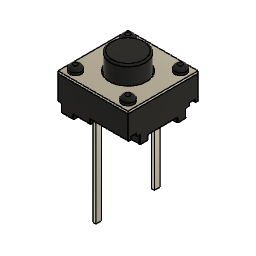
6x6x5 (Autodesk Fusion 360 design; units mm, degrees)
Autodesk Fusion 360 part; units mm, degrees
note: some values were not read from the file. Chosen so that the rebuilt part matches the saved one: which pieces of a blend or face edit are solid.
sketch "Sketch1" plane through (0, 0, 0) normal (0, 0, 1) x (1, 0, 0)
  line L0 (3, -3) -> (-3, -3)
  line L1 (-3, -3) -> (-3, 3)
  line L2 (-3, 3) -> (3, 3)
  line L3 (3, 3) -> (3, -3)
  line L4 (3, -3) -> (-3, 3) construction
  line L5 (-3, -3) -> (3, 3) construction
  dimension "d1" = 6
  dimension "d2" = 6
  constraint horizontal L0
  constraint perpendicular L0 L1
  constraint parallel L0 L2
  constraint parallel L1 L3
  constraint coincident L4 origin
  constraint coincident L5 origin
  measures "d1" distance of L1.end L2.end
  measures "d2" distance of L0.end L1.end
extrude "Extrude1" add sketch "Sketch1" along normal blind 2.8 makes body 1
extrude "Extrude2" add 1 faces at (-1, -1, 2.8) along direction (0, 0, 1) blind 0.2 separate body on bodies 1 makes body 2
sketch "Sketch2" plane through (0, 0, 3) normal (0, 0, 1) x (-1, 0, 0)
  line L0 (-3, -3) -> (3, -3)
  line L1 (3, -3) -> (3, 3)
  line L2 (3, 3) -> (-3, 3)
  line L3 (-3, 3) -> (-3, -3)
  circle A0 centre (2.25, -2.25) radius 0.5
  circle A1 centre (0, 0) radius 1.5
  circle A2 centre (0, 0) radius 1.6
  dimension "d7" = 1
  dimension "d8" = 0.75
  dimension "d9" = 0.75
  dimension "d10" = 3
  dimension "d23" = 3.2
  constraint coincident A1.centre A2.centre
  constraint concentric A1 A2
  measures "d7" diameter of A0
  measures "d8" distance of L0 A0.centre
  measures "d9" distance of L1 A0.centre
  measures "d10" diameter of A1
  measures "d23" diameter of A2
extrude "Extrude3" add sketch "Sketch2" along normal blind 0.5 contours A0 bodies 2
extrude "Extrude4" add sketch "Sketch2" along normal blind 1.5 contours A1 bodies 2
fillet "Fillet1" radius 0.3 1 edges at (-1.7838, 2.4308, 3.5) on bodies 2
mirror "Mirror1" about plane through (0, 0, 0) normal (1, 0, 0) of "Extrude3", "Fillet1"
mirror "Mirror2" about plane through (0, 0, 0) normal (0, 1, 0) of "Extrude3", "Fillet1", "Mirror1"
fillet "Fillet2" radius 0.15 1 edges at (1.3985, 0.5424, 4.5) on bodies 2
extrude "Extrude5" cut sketch "Sketch2" against normal blind 0.2 contours A2 bodies 2 makes body 3 at (-0.0399, 2.5318, 2.8)
sketch "Sketch3" plane through (3, 0, 0) normal (1, 0, 0) x (0, 1, 0)
  line L0 (-3, 0) -> (3, 0)
  line L1 (3, 0) -> (3, 2.8)
  line L2 (3, 2.8) -> (-3, 2.8)
  line L3 (-3, 2.8) -> (-3, 0)
  line L4 (-2, 0) -> (-1.25, 0)
  line L5 (-1.25, 0) -> (-1.25, 0.75)
  line L6 (-1.25, 0.75) -> (-2, 0.75)
  line L7 (-2, 0.75) -> (-2, 0)
  line L8 (-2.75, 0.75) -> (-2.25, 0.75)
  line L9 (-2.25, 0.75) -> (-2.25, 1)
  line L10 (-2.25, 1) -> (-2.75, 1)
  line L11 (-2.75, 1) -> (-2.75, 0.75)
  line L12 (-2, 0.75) -> (-3, 0.75)
  line L13 (2, 0) -> (1.25, 0)
  line L14 (1.25, 0) -> (1.25, 0.75)
  line L15 (1.25, 0.75) -> (2, 0.75)
  line L16 (2, 0.75) -> (2, 0)
  line L17 (-1.25, 0.75) -> (1.25, 0.75)
  line L18 (1.25, 0.75) -> (1.25, 0.375)
  line L19 (1.25, 0.375) -> (-1.25, 0.375)
  line L20 (-1.25, 0.375) -> (-1.25, 0.75)
  line L21 (2, 0.75) -> (3, 0.75)
  line L22 (2.75, 0.75) -> (2.25, 0.75)
  line L23 (2.25, 0.75) -> (2.25, 1)
  line L24 (2.25, 1) -> (2.75, 1)
  line L25 (2.75, 1) -> (2.75, 0.75)
  dimension "d26" = 0.75
  dimension "d27" = 0.75
  dimension "d28" = 1
  dimension "d29" = 0.5
  dimension "d30" = 0.25
  dimension "d31" = 0.25
  dimension "d32" = 0.75
  dimension "d33" = 0.75
  dimension "d34" = 1
  dimension "d35" = 0.5
  dimension "d36" = 0.25
  dimension "d37" = 0.25
  constraint horizontal L4
  constraint vertical L5
  constraint horizontal L6
  constraint vertical L7
  constraint coincident L0 L4.start
  constraint horizontal L8
  constraint vertical L9
  constraint horizontal L10
  constraint vertical L11
  constraint coincident L3 L12.end
  constraint perpendicular L3 L12
  constraint horizontal L13
  constraint vertical L14
  constraint horizontal L15
  constraint vertical L16
  constraint coincident L0 L13.start
  constraint horizontal L17
  constraint vertical L18
  constraint horizontal L19
  constraint vertical L20
  constraint midpoint L14 L18.end
  constraint coincident L1 L21.end
  constraint perpendicular L1 L21
  constraint horizontal L22
  constraint vertical L23
  constraint horizontal L24
  constraint vertical L25
  constraint coincident L21 L22.start
  measures "d26" distance of L4.start L4.end
  measures "d27" distance of L4.start L6.end
  measures "d28" distance of L3 L7
  measures "d29" distance of L8.start L8.end
  measures "d30" distance of L8.start L10.end
  measures "d31" distance of L3 L11
  measures "d32" distance of L13.start L13.end
  measures "d33" distance of L13.start L15.end
  measures "d34" distance of L1 L16
  measures "d35" distance of L22.start L22.end
  measures "d36" distance of L22.start L24.end
  measures "d37" distance of L1 L25
extrude "Extrude6" cut sketch "Sketch3" against normal blind 3.25 contours L0 L3 L7 L8 L12 | L0 L5 L14 L19 | L8 L9 L10 L11 L12 | L0 L1 L16 L21 L22 | L21 L22 L23 L24 L25 bodies 1
sketch "Sketch4" plane through (-3, 0, 0) normal (-1, 0, 0) x (0, -1, 0)
  line L0 (-3, 0) -> (3, 0)
  line L1 (3, 0) -> (3, 2.8)
  line L2 (3, 2.8) -> (-3, 2.8)
  line L3 (-3, 2.8) -> (-3, 0)
  line L4 (-3, 0) -> (-1.5, 0)
  line L5 (-1.5, 0) -> (-1.5, 0.75)
  line L6 (-1.5, 0.75) -> (-3, 0.75)
  line L7 (-3, 0.75) -> (-3, 0)
  line L8 (3, 0) -> (1.5, 0)
  line L9 (1.5, 0) -> (1.5, 0.75)
  line L10 (1.5, 0.75) -> (3, 0.75)
  line L11 (3, 0.75) -> (3, 0)
  dimension "d42" = 1.5
  dimension "d43" = 0.75
  dimension "d44" = 1.5
  dimension "d45" = 0.75
  constraint horizontal L4
  constraint vertical L5
  constraint horizontal L6
  constraint vertical L7
  constraint coincident L0.start L3.end
  constraint horizontal L8
  constraint vertical L9
  constraint horizontal L10
  constraint vertical L11
  constraint coincident L0.end L1.start
  measures "d42" distance of L0.start L4.end
  measures "d43" distance of L0.start L6.end
  measures "d44" distance of L0.end L8.end
  measures "d45" distance of L0.end L10.end
extrude "Extrude7" cut 1 faces at (-0.25, 0.4167, 0.125) along direction (-1, 0, 0) blind 4 on bodies 1 bodies 1
extrude "Extrude8" cut sketch "Sketch4" against normal blind 0.3 contours L0 L3 L4 L5 L6 L7 | L0 L1 L8 L9 L10 L11 bodies 1
sketch "Sketch5" plane through (0, 0, 0) normal (0, 0, -1) x (1, 0, 0)
  line L0 (-2.7, -1.5) -> (-2.7, -3)
  line L1 (-2.7, -3) -> (-0.25, -3)
  line L2 (-0.25, -3) -> (-0.25, -2)
  line L3 (-0.25, -2) -> (3, -2)
  line L4 (3, -2) -> (3, -1.25)
  line L5 (3, -1.25) -> (-3, -1.25)
  line L6 (-3, -1.25) -> (-3, -1.5)
  line L7 (-3, -1.5) -> (-2.7, -1.5)
  line L8 (-2.7, -3) -> (-1.7, -3)
  line L9 (-1.7, -3) -> (-1.7, -1.5)
  line L10 (-1.7, -1.5) -> (-2.7, -1.5)
  line L11 (-2.7, -1.5) -> (-2.7, -3)
  line L12 (3, -1.25) -> (2, -1.25)
  line L13 (2, -1.25) -> (2, -2)
  line L14 (2, -2) -> (3, -2)
  line L15 (3, -2) -> (3, -1.25)
  line L16 (-1.7, -1.5) -> (2, -1.5)
  dimension "d48" = 1
  dimension "d49" = 1.5
  dimension "d50" = 1
  dimension "d51" = 0.75
  constraint horizontal L8
  constraint vertical L9
  constraint horizontal L10
  constraint vertical L11
  constraint coincident L0.end L1.start
  constraint horizontal L12
  constraint vertical L13
  constraint horizontal L14
  constraint vertical L15
  constraint coincident L4.end L5.start
  constraint coincident L13 L16.end
  constraint perpendicular L13 L16
  measures "d48" distance of L0.end L8.end
  measures "d49" distance of L0.end L0.start
  measures "d50" distance of L4.end L12.end
  measures "d51" distance of L4.end L3.end
extrude "Extrude9" cut sketch "Sketch5" against normal blind 0.375 contours L1 L2 L3 L9 L13 L16 bodies 1
mirror "Mirror3" about plane through (0, 0, 0) normal (0, 1, 0) of "Extrude9"
sketch "Sketch6" plane through (0, 0, 0.375) normal (0, 0, -1) x (1, 0, 0)
  line L0 (3, -1.25) -> (3, 1.25)
  line L1 (3, 1.25) -> (-3, 1.25)
  line L2 (-3, 1.25) -> (-3, -1.25)
  line L3 (-3, -1.25) -> (3, -1.25)
  line L4 (1.45, 1.1) -> (2.85, 1.1)
  line L5 (2.85, 1.1) -> (2.85, -1.1)
  line L6 (2.85, -1.1) -> (1.45, -1.1)
  line L7 (1.45, -1.1) -> (1.45, 1.1)
  line L8 (1.45, 1.1) -> (2.85, -1.1) construction
  line L9 (2.85, 1.1) -> (1.45, -1.1) construction
  point P0 (2.15, 0)
  dimension "d56" = 1.4
  dimension "d57" = 2.2
  dimension "d58" = 0.15
  constraint horizontal L4
  constraint perpendicular L4 L5
  constraint parallel L4 L6
  constraint parallel L5 L7
  constraint coincident L8 P0
  constraint coincident L9 P0
  measures "d56" distance of L5.end L6.end
  measures "d57" distance of L4.end L5.end
  measures "d58" distance of L0 L5
extrude "Extrude10" cut sketch "Sketch6" against normal blind 0.15 contours L4 L5 L6 L7 bodies 1
mirror "Mirror4" about plane through (0, 0, 0) normal (1, 0, 0) of "Extrude10"
sketch "Sketch7" plane through (0, 0, 1) normal (0, 0, -1) x (1, 0, 0)
  line L0 (3, 2.25) -> (3, 2.75)
  line L1 (3, 2.75) -> (-0.25, 2.75)
  line L2 (-0.25, 2.75) -> (-0.25, 2.25)
  line L3 (-0.25, 2.25) -> (3, 2.25)
  line L4 (-0.25, 2.75) -> (0, 2.75)
  line L5 (0, 2.75) -> (0, 2.25)
  line L6 (0, 2.25) -> (-0.25, 2.25)
  line L7 (-0.25, 2.25) -> (-0.25, 2.75)
  dimension "d63" = 0.25
  constraint horizontal L4
  constraint vertical L5
  constraint horizontal L6
  constraint vertical L7
  constraint coincident L3 L5.end
  constraint coincident L1.end L2.start
  measures "d63" distance of L1.end L4.end
extrude "Extrude11" add sketch "Sketch7" along normal blind 8 contours L1 L2 L3 L4 L5 L6 L7 bodies 1
mirror "Mirror5" about plane through (0, 0, 0) normal (0, 1, 0) of "Extrude11"
fillet "Fillet3" radius 0.05 31 edges at (0, -1.25, 0.375) (0, 1.25, 0.375) (3, 0, 0.375) (3, -1.25, 0.1875) (3, -2, 0.375) (3, 1.25, 0.1875) (3, 2, 0.375) (1.5, -2.25, 0.75) (1.5, -2.75, 0.75) (1.375, -3, 0.75) (1.375, 3, 0.75) (1.5, 2.75, 0.75) (1.5, 2.25, 0.75) (-0.25, -3, 0.5625) (-0.975, -3, 0.375) (-1.7, -3, 0.1875) (-2.2, -3, 0) (-0.25, 3, 0.5625) (-0.975, 3, 0.375) (-1.7, 3, 0.1875) (-2.2, 3, 0) (-3, 1.5, 0.375) (-3, -1.25, 0.1875) (-3, 1.25, 0.1875) (-3, -1.5, 0.375) (2, -1.5, 0.1875) (2.5, -2, 0) (2, 1.5, 0.1875) (2.5, 2, 0) (-1.7, 1.5, 0.1875) (-1.7, -1.5, 0.1875) on bodies 1
